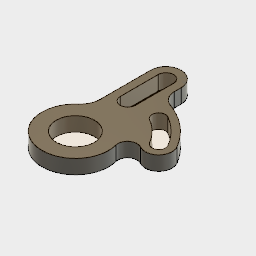
!-1 (Autodesk Fusion 360 archive; units mm, degrees)
design "模型1"
Autodesk Fusion 360 part; units mm, degrees
sketch "草图1" plane through (0, 0, 0) normal (0, 1, 0) x (1, 0, 0)
  circle A0 centre (-40.3928, -121.0386) radius 20
  line L0 (-48.3928, -26.0386) -> (-48.3928, -66.0386)
  line L1 (-32.3928, -26.0386) -> (-32.3928, -66.0386)
  line L2 (-56.3928, -26.0386) -> (-56.3928, -79.0062)
  arc A1 (-63.5162, -94.7649) -> (-56.3928, -79.0062) centre (-77.3855, -79.0062) ccw
  line L3 (-24.3928, -26.0386) -> (-24.3928, -33.3574)
  arc A2 (21.095, -85.5386) -> (-4.8928, -59.5508) centre (-40.3928, -121.0386) ccw
  arc A3 (8.9707, -92.5386) -> (-11.8928, -71.6752) centre (-40.3928, -121.0386) ccw
  arc A4 (8.1383, -101.2233) -> (-6.4767, -112.3959) centre (3.2137, -109.9266) ccw
  line L4 (-28.27, -15.5965) -> (18.7059, -70.1334)
  arc A5 (27.1572, -82.0386) -> (-14.3928, -47.4995) centre (-40.3928, -121.0386) ccw
  arc A6 (-7.6667, -66.0386) -> (-8.3928, -65.613) centre (-40.3928, -121.0386) ccw
  line L5 (-8.6385, -66.0386) -> (-8.3928, -65.613)
  arc A7 (-4.8928, -59.5508) -> (-11.8928, -71.6752) centre (-8.3928, -65.613) ccw
  line L6 (4.5071, -66.0386) -> (4.9473, -66.0386)
  arc A8 (8.1383, -101.2233) -> (27.1572, -82.0386) centre (15.0328, -89.0386) ccw
  arc A9 (8.9707, -92.5386) -> (21.095, -85.5386) centre (15.0328, -89.0386) ccw
  arc A10 (-63.5162, -94.7649) -> (-6.4767, -112.3959) centre (-40.3928, -121.0386) ccw
  arc A11 (-48.3928, -66.0386) -> (-32.3928, -66.0386) centre (-40.3928, -66.0386) ccw
  arc A12 (-24.3928, -26.0386) -> (-56.3928, -26.0386) centre (-40.3928, -26.0386) ccw
  arc A13 (-32.3928, -26.0386) -> (-48.3928, -26.0386) centre (-40.3928, -26.0386) ccw
  arc A14 (-24.3928, -33.3574) -> (-14.3928, -47.4995) centre (-9.3928, -33.3574) ccw
  dimension "d3" = 40
  dimension "d4" = 70
  dimension "d5" = 95
  dimension "d6" = 16
  dimension "d7" = 32
  dimension "d9" = 16
  dimension "d11" = 142
  dimension "d12" = 114
  dimension "d15" = 14
  dimension "d16" = 14
  dimension "d17" = 28
  dimension "d18" = 20
  dimension "d19" = 156
  dimension "d20" = 30
  measures "d3" diameter of A0
  measures "d4" diameter of A10
  measures "d5" distance of A0.centre A12.centre
  measures "d6" diameter of A13
  measures "d7" diameter of A12
  measures "d9" diameter of A11
  measures "d11" diameter of A2
  measures "d12" diameter of A3
  measures "d15" diameter of A7
  measures "d16" diameter of A9
  measures "d17" diameter of A8
  measures "d18" diameter of A4
  measures "d19" diameter of A5
  measures "d20" diameter of A14
sketch "草图2" plane through (11.3081, 0, 26.2456) normal (0, 1, 0) x (1, 0, 0)
extrude "拉伸1" add sketch "草图1" along normal blind 10 contours L2 A1 L3 A4 A5 A8 A10 A12 A14
sketch "草图3" plane through (0, 0, 0) normal (1, 0, 0) x (0, 0, -1)
extrude "拉伸2" add 1 faces at (-26.185, 0, 82.3657) along direction (0, -1, 0) blind 5
sketch "草图4" plane through (0, 10, 0) normal (0, 1, 0) x (-1, 0, 0)
  circle A0 centre (40.3928, 121.0386) radius 20
  arc A1 (32.3928, 26.0386) -> (48.3928, 26.0386) centre (40.3928, 26.0386) ccw
  line L0 (32.3928, 26.0386) -> (32.3928, 66.0386)
  arc A2 (48.3928, 66.0386) -> (32.3928, 66.0386) centre (40.3928, 66.0386) ccw
  line L1 (48.3928, 66.0386) -> (48.3928, 26.0386)
  arc A3 (-8.9707, 92.5386) -> (-21.095, 85.5386) centre (-15.0328, 89.0386) ccw
  arc A4 (-8.9707, 92.5386) -> (11.8928, 71.6752) centre (40.3928, 121.0386) ccw
  arc A5 (4.8928, 59.5508) -> (11.8928, 71.6752) centre (8.3928, 65.613) ccw
  arc A6 (-21.095, 85.5386) -> (4.8928, 59.5508) centre (40.3928, 121.0386) ccw
  arc A7 (24.3928, 26.0386) -> (56.3928, 26.0386) centre (40.3928, 26.0386) ccw
  line L2 (56.3928, 26.0386) -> (56.3928, 79.0062)
  arc A8 (63.5162, 94.7649) -> (56.3928, 79.0062) centre (77.3855, 79.0062) ccw
  arc A9 (63.5162, 94.7649) -> (6.4767, 112.3959) centre (40.3928, 121.0386) ccw
  arc A10 (-8.1383, 101.2233) -> (6.4767, 112.3959) centre (-3.2137, 109.9266) ccw
  arc A11 (-8.1383, 101.2233) -> (-27.1572, 82.0386) centre (-15.0328, 89.0386) ccw
  arc A12 (-27.1572, 82.0386) -> (14.3928, 47.4995) centre (40.3928, 121.0386) ccw
  arc A13 (24.3928, 33.3574) -> (14.3928, 47.4995) centre (9.3928, 33.3574) ccw
  line L3 (24.3928, 33.3574) -> (24.3928, 26.0386)
